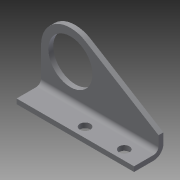
# Autodesk Inventor part: Flange Bearing Mount Tower
Saved by Autodesk Inventor 2013 (Build 170138000, 138)
## iProperties
Created: 2013-01-21
Part Number: Flange Bearing Mount Tower
Material: Generic
Document SubType Name: Sheet Metal
Designer: actoennies
Density: 1 g/cm^3
Sheet Metal Rule: Default
Mass: 8.97134 g
Surface Area: 68.258 cm^2
Volume: 8.97134 cm^3
Author: actoennies
Autodesk Inventor part; units mm, degrees
ref_plane "YZ Plane" through (0, 0, 0) normal (1, 0, 0) x (0, 1, 0)
ref_plane "XZ Plane" through (0, 0, 0) normal (0, 1, 0) x (-1, 0, 0)
ref_plane "XY Plane" through (0, 0, 0) normal (0, 0, 1) x (1, 0, 0)
sketch "Sketch1" plane through (0, 0, 0) normal (0, 1, 0) x (-1, 0, 0)
  line L0 (0, 0) -> (-76.2, 0)
  line L1 (-76.2, 0) -> (-76.2, 12.7)
  line L2 (-76.2, 12.7) -> (-38.1, 12.7)
  line L3 (0, 12.7) -> (0, 0)
  line L4 (0, 0) -> (-12.7, 0)
  circle A0 centre (-38.1, 6.35) radius 3.3782
  circle A1 centre (-63.5, 6.35) radius 3.3782
  line L5 (-38.1, 12.7) -> (0, 12.7)
  dimension "d0" = 12.7
  dimension "d2" = 76.2
  dimension "d5" = 6.7564
  dimension "d7" = 6.7564
  dimension "d8" = 6.35
  dimension "d9" = 38.1
  dimension "d10" = 6.35
  dimension "d11" = 12.7
  dimension "d12" = 38.1
  measures "d0" distance between parallel lines of L0 L2
  measures "d2" distance of L1.end L3.start
  measures "d5" diameter of A0
  measures "d7" diameter of A1
  measures "d8" distance from line of L0 A0.centre
  measures "d9" distance from line of L3 A0.centre
  measures "d10" distance from line of L2 A1.centre
  measures "d11" distance from line of L1 A1.centre
  measures "d12" distance of L1.end L2.end
extrude "Plate2" add sketch "Sketch1" along normal blind 3.175
sketch "Sketch5" plane through (0, 6.35, -3.175) normal (0, 0, -1) x (-1, 0, 0)
  line L0 (-76.2, 0) -> (0, 0)
  line L1 (0, 0) -> (0, 38.1)
  line L2 (0, 38.1) -> (-76.2, 38.1)
  line L3 (-76.2, 38.1) -> (-76.2, 0)
  constraints: 6 end point, 1 horizontal, 1 perpendicular, 1 vertical
edge flange "Flange2" height 44.45 angle 90 thickness 3.175 bend radius 3.175 thickness toward (0, 0, -1) relief straight relief width 3.175 relief depth 1.5875 edges at (38.1, 3.175, 0) wall of the first edge with corners at (76.2, 6.35, -3.175) (0, 6.35, -3.175) (0, 44.45, -3.175) (76.2, 44.45, -3.175)
bend "Bend2"
corner "Corner2"
sketch "Sketch6" plane through (0, 44.45, -3.175) normal (0, 0, 1) x (1, 0, 0)
  line L0 (0, -38.1) -> (76.2, -38.1) projected
  line L1 (76.2, 0) -> (76.2, -38.1) projected
  line L2 (76.2, 0) -> (0, 0) projected
  line L3 (0, 0) -> (0, -38.1) projected
  circle A0 centre (19.05, -19.05) radius 14.2875
  arc A1 (29.0088, -2.8104) -> (0, -19.05) centre (19.05, -19.05) ccw
  line L4 (76.2, -31.75) -> (29.0088, -2.8104)
  point P0 (0, -44.45)
  dimension "d50" = 28.575
  dimension "d51" = 19.05
  dimension "d52" = 19.05
  dimension "d53" = 6.35
  constraints: 2 centre point, 2 end point, 2 point on circle, 2 tangent, 1 coincident, 1 midpoint, 1 point on line
  measures "d50" diameter of A0
  measures "d51" distance from line of L2 A0.centre
  measures "d52" distance from line of L3 A0.centre
  measures "d53" distance of L0.end L4.start
extrude "Cut3" cut sketch "Sketch6" against normal blind 3.175 contours L3 L2 A1 | L4 A1 L2 L1 | A0
equation "\"d54\" = Thickness"
equation "\"d40\" = BendReliefWidth"
equation "\"d41\" = BendReliefDepth"
equation "\"d42\" = MinimumRemnant"
equation "\"d43\" = BendRadius"
equation "\"d46\" = BendRadius"
equation "\"d47\" = CornerReliefSize"
equation "\"d48\" = GapSize"
equation "\"d49\" = JacobiRadiusSize"
equation "\"BendRadius\" = Thickness"
equation "\"BendReliefWidth\" = Thickness"
equation "\"BendReliefDepth\" = 0.5 * Thickness"
equation "\"CornerReliefSize\" = 4 * Thickness"
equation "\"MinimumRemnant\" = 2 * Thickness"
equation "\"TransitionRadius\" = BendRadius"
equation "\"JacobiRadiusSize\" = BendRadius"
equation "\"GapSize\" = Thickness"
equation "\"d18\" = BendRadius"
equation "\"d19\" = BendRadius"
equation "\"Thickness\" = 3.175"
body "Solid2"
